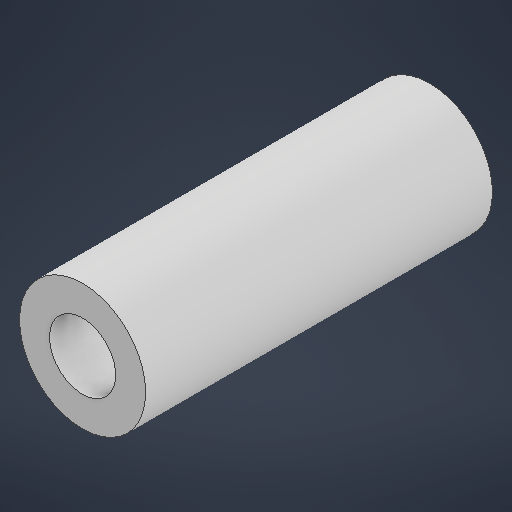
# Autodesk Inventor part: ADC_Zylinder
Saved by Autodesk Inventor 2026.2 (Build 302298000, 298)
## iProperties
Created: 2026-01-10
Part Number: ADC_Zylinder
Material: Generisch
Document SubType Name: Modeling
Designer: Alex
Density: 1 g/cm^3
Appearance: Vorgabe
Author: Alex
Autodesk Inventor part; units mm, degrees
ref_plane "YZ Plane" through (0, 0, 0) normal (1, 0, 0) x (0, 1, 0)
ref_plane "XZ Plane" through (0, 0, 0) normal (0, 1, 0) x (-1, 0, 0)
ref_plane "XY Plane" through (0, 0, 0) normal (0, 0, 1) x (1, 0, 0)
sketch "Skizze1" plane through (0, 0, 0) normal (0, 1, 0) x (-1, 0, 0)
  circle A0 centre (0, 0) radius 1.05
  circle A1 centre (0, 0) radius 2
  dimension "d1" = 2.1
  dimension "d2" = 4
  constraints: 2 centre point, 2 coincident
  measures "d1" diameter of A0
  measures "d2" diameter of A1
extrude "Extrusion1" add sketch "Skizze1" along normal blind 11
